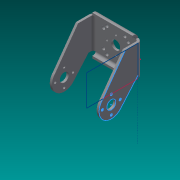
# Autodesk Inventor part: 45angle
Saved by Autodesk Inventor 2013 SP2 (Build 170200200, 200)
## iProperties
Created: 2014-11-26
Part Number: 45angle
Material: Generic
Document SubType Name: Sheet Metal
Designer: Master
Density: 1 g/cm^3
Sheet Metal Rule: Default_mm
Author: Master
Autodesk Inventor part; units mm, degrees
ref_plane "YZ Plane" through (0, 0, 0) normal (1, 0, 0) x (0, 1, 0)
ref_plane "XZ Plane" through (0, 0, 0) normal (0, 1, 0) x (-1, 0, 0)
ref_plane "XY Plane" through (0, 0, 0) normal (0, 0, 1) x (1, 0, 0)
sketch "Sketch1" plane through (0, 0, 0) normal (0, 1, 0) x (-1, 0, 0)
  circle A0 centre (0, 0) radius 4
  circle A1 centre (0, 8) radius 1
  circle A2 centre (8, 0) radius 1
  circle A3 centre (-8, 0) radius 1
  circle A4 centre (0, -8) radius 1
  circle A5 centre (-11, 8) radius 1.5
  circle A6 centre (11, -8) radius 1.5
  circle A7 centre (11, 8) radius 1.5
  circle A8 centre (-11, -8) radius 1.5
  line L0 (-18, 13.75) -> (18, 13.75)
  line L1 (18, 13.75) -> (18, -13.75)
  line L2 (18, -13.75) -> (-18, -13.75)
  line L3 (-18, -13.75) -> (-18, 13.75)
  line L4 (-17, 13.75) -> (19, -13.75) construction
  line L5 (19, 13.75) -> (-17, -13.75) construction
  point P0 (0, 0)
  dimension "d0" = 36
  dimension "d1" = 27.5
  measures "d0" distance of L1.end L2.end
  measures "d1" distance of L0.end L1.end
extrude "Plate1" add sketch "Sketch1" along normal blind 2
sketch "Sketch4" plane through (20, -2, 13.75) normal (1, 0, 0) x (0, 1, 0)
  line L0 (0, -27.5) -> (0, 0)
  line L1 (0, 0) -> (-46, 0)
  line L2 (-46, 0) -> (-46, -27.5)
  line L3 (-46, -27.5) -> (0, -27.5)
  constraints: 6 end point, 1 horizontal, 1 perpendicular, 1 vertical
edge flange "Flange3" height 50 angle 90 thickness 2 bend radius 2 thickness toward (1, 0, 0) relief straight relief width 2 relief depth 1 edges at (18, 0, 0) wall of the first edge with corners at (20, -2, -13.75) (20, -2, 13.75) (20, -48, 13.75) (20, -48, -13.75)
bend "Bend3"
corner "Corner3"
sketch "Sketch5" plane through (-20, -2, -13.75) normal (-1, 0, 0) x (0, -1, 0)
  line L0 (0, 27.5) -> (0, 0)
  line L1 (0, 0) -> (46, 0)
  line L2 (46, 0) -> (46, 27.5)
  line L3 (46, 27.5) -> (0, 27.5)
  constraints: 6 end point, 1 horizontal, 1 perpendicular, 1 vertical
edge flange "Flange4" height 50 angle 90 thickness 2 bend radius 2 thickness toward (-1, 0, 0) relief straight relief width 2 relief depth 1 edges at (-18, 0, 0) wall of the first edge with corners at (-20, -2, 13.75) (-20, -2, -13.75) (-20, -48, -13.75) (-20, -48, 13.75)
bend "Bend4"
corner "Corner4"
sketch "Sketch6" plane through (22, -48, 13.75) normal (1, 0, 0) x (0, 0, -1)
  line L0 (27.5, 46) -> (0, 46) projected
  line L1 (0, 0) -> (0, 46) projected
  line L2 (13.75, 46) -> (78.0909, 46) construction
  circle A0 centre (27.7916, 21.9584) radius 1
  circle A1 centre (35.7916, 29.9584) radius 1
  circle A2 centre (43.7916, 21.9584) radius 1
  circle A3 centre (35.7916, 13.9584) radius 1
  circle A4 centre (35.7916, 21.9584) radius 4
  arc A5 (28.0135, 14.1802) -> (42.3794, 30.7675) centre (35.7916, 21.9584) ccw
  line L3 (43.5698, 29.7365) -> (24.7916, 46)
  line L4 (28.0135, 14.1802) -> (0, 34.3911)
  line L5 (24.7916, 46) -> (27.5, 46)
  line L6 (24.7916, 46) -> (0, 46)
  line L7 (0, 46) -> (0, 34.3911)
  line L8 (27.5, 46) -> (27.5, 0) projected
  line L9 (0, 34.3911) -> (0, 0)
  line L10 (27.5, 0) -> (0, 0)
  line L11 (27.5, 0) -> (27.5, 14.5506)
  line L12 (27.5, 14.5506) -> (0, 34.3911)
  point P0 (13.75, 48)
  constraints: 20 end point, 6 centre point, 5 point on line, 4 collinear, 3 point on circle, 1 horizontal, 1 midpoint, 1 parallel, 1 perpendicular
sheet face with bend "Face2" sketch "Sketch6" thickness 2 toward (-1, 0, 0) bend radius 2 relief straight relief width 2 relief depth 1 contours L3 L8 A0 L4 L1 L0 | L3 A5 L4 L8 A0
bend "Bend5"
extrude "Cut1" cut sketch "Sketch6" against normal blind 2 contours L4 L8 L10 L1
sketch "Sketch7" plane through (0, 2, 0) normal (0, 1, 0) x (1, 0, 0)
  circle A0 centre (0, 0) radius 4 projected
  circle A1 centre (-11, -8) radius 1.5 projected
  circle A2 centre (11, -8) radius 1.5 projected
  circle A3 centre (-11, 8) radius 1.5 projected
  circle A4 centre (11, 8) radius 1.5 projected
  circle A5 centre (0, -8) radius 1 projected
  circle A6 centre (-8, 0) radius 1 projected
  circle A7 centre (8, 0) radius 1 projected
  circle A8 centre (0, 8) radius 1 projected
  line L0 (18, 11.75) -> (-18, 11.75) projected
  line L1 (-18, -13.75) -> (-18, 13.75) projected
  line L2 (-18, -11.75) -> (18, -11.75) projected
  line L3 (18, 13.75) -> (18, -13.75) projected
  line L4 (0, -11.75) -> (0, 11.75)
  constraints: 2 end point, 2 midpoint
ref_plane "Work Plane1" through (0, 2, 11.75) normal (1, 0, 0) x (0, 0, -1)
mirror "Mirror1" about plane through (0, 2, 11.75) normal (1, 0, 0) of "Flange3", "Face2"
sketch "Sketch8" plane through (-22, -48, -13.75) normal (-1, 0, 0) x (0, 0, 1)
  line L0 (0, 0) -> (0, 14.5506) projected
  line L1 (27.5, 0) -> (0, 0) projected
  line L2 (27.5, 46) -> (27.5, 0) projected
  line L3 (-0.5135, 14.1802) -> (27.5, 34.3911) projected
  line L4 (0, 14.5506) -> (27.5, 34.3911)
  line L5 (27.5, 34.3911) -> (27.5, 0)
  line L6 (0, 0) -> (0, 14.5506)
  line L7 (0, 0) -> (27.5, 0)
  point P0 (13.75, 48)
  constraints: 8 end point, 4 collinear
extrude "Cut2" cut sketch "Sketch8" against normal blind 2
sketch "Sketch9" plane through (0, 2, 0) normal (0, 1, 0) x (1, 0, 0)
  circle A0 centre (0, 0) radius 4 projected
  circle A1 centre (-11, -8) radius 1.5 projected
  circle A2 centre (11, -8) radius 1.5 projected
  circle A3 centre (-11, 8) radius 1.5 projected
  circle A4 centre (11, 8) radius 1.5 projected
  circle A5 centre (0, -8) radius 1 projected
  circle A6 centre (-8, 0) radius 1 projected
  circle A7 centre (8, 0) radius 1 projected
  circle A8 centre (0, 8) radius 1 projected
  line L0 (18, 11.75) -> (-18, 11.75) projected
  line L1 (-18, -13.75) -> (-18, 13.75) projected
  line L2 (-18, -11.75) -> (18, -11.75) projected
  line L3 (18, 13.75) -> (18, -13.75) projected
  line L4 (0, -4) -> (0, 4)
  constraints: 2 end point, 2 point on circle, 1 parallel
sketch "Sketch10" plane through (0, 2, 0) normal (0, 1, 0) x (1, 0, 0)
  circle A0 centre (0, 0) radius 4 projected
  circle A1 centre (-11, -8) radius 1.5 projected
  circle A2 centre (11, -8) radius 1.5 projected
  circle A3 centre (-11, 8) radius 1.5 projected
  circle A4 centre (11, 8) radius 1.5 projected
  circle A5 centre (0, -8) radius 1 projected
  circle A6 centre (-8, 0) radius 1 projected
  circle A7 centre (8, 0) radius 1 projected
  circle A8 centre (0, 8) radius 1 projected
  line L0 (18, 11.75) -> (-18, 11.75) projected
  line L1 (-18, -13.75) -> (-18, 13.75) projected
  line L2 (-18, -11.75) -> (18, -11.75) projected
  line L3 (18, 13.75) -> (18, -13.75) projected
sketch "Sketch11" plane through (0, 2, 0) normal (0, 1, 0) x (1, 0, 0)
  circle A0 centre (0, 0) radius 4 projected
  circle A1 centre (11, 8) radius 1.5 projected
  circle A2 centre (-11, 8) radius 1.5 projected
  circle A3 centre (11, -8) radius 1.5 projected
  circle A4 centre (-11, -8) radius 1.5 projected
  circle A5 centre (-11, 8) radius 1.5
  circle A6 centre (11, 8) radius 1.5
  circle A7 centre (11, -8) radius 1.5
  circle A8 centre (-11, -8) radius 1.5
  line L0 (8, -11) -> (-8, 11) construction
  line L1 (-8, -11) -> (8, 11) construction
  circle A9 centre (-8, 11) radius 1.5
  circle A10 centre (8, 11) radius 1.5
  circle A11 centre (8, -11) radius 1.5
  circle A12 centre (-8, -11) radius 1.5
  dimension "d62" = 16
  dimension "d63" = 22
  dimension "d64" = 3
  dimension "d65" = 3
  dimension "d66" = 3
  dimension "d67" = 3
  constraints: 8 centre point, 8 coincident, 4 end point, 2 midpoint, 1 concentric
  measures "d62" distance of L0.end L1.end
  measures "d63" distance of L1.start L0.end
  measures "d64" diameter of A9
  measures "d65" diameter of A10
  measures "d66" diameter of A11
  measures "d67" diameter of A12
extrude "Cut3" cut sketch "Sketch11" against normal blind 2 contours A9 | A10 | A11 | A12
sketch "Sketch12" plane through (-18, -2, 15.75) normal (0, 0, 1) x (1, 0, 0)
  line L0 (36, 0) -> (0, 0)
  line L1 (0, 0) -> (0, -1)
  line L2 (0, -1) -> (36, -1)
  line L3 (36, -1) -> (36, 0)
  constraints: 6 end point, 1 horizontal, 1 perpendicular, 1 vertical
edge flange "Flange5" height 5 angle 90 thickness 2 bend radius 2 thickness toward (0, 0, 1) relief straight relief width 2 relief depth 1 edges at (0, 0, 13.75) wall of the first edge with corners at (18, -2, 15.75) (-18, -2, 15.75) (-18, -3, 15.75) (18, -3, 15.75)
bend "Bend6"
corner "Corner5"
sketch "Sketch13" plane through (18, -2, -15.75) normal (0, 0, -1) x (-1, 0, 0)
  line L0 (36, 0) -> (0, 0)
  line L1 (0, 0) -> (0, -1)
  line L2 (0, -1) -> (36, -1)
  line L3 (36, -1) -> (36, 0)
  constraints: 6 end point, 1 horizontal, 1 perpendicular, 1 vertical
edge flange "Flange6" height 5 angle 90 thickness 2 bend radius 2 thickness toward (0, 0, -1) relief straight relief width 2 relief depth 1 edges at (0, 0, -13.75) wall of the first edge with corners at (-18, -2, -15.75) (18, -2, -15.75) (18, -3, -15.75) (-18, -3, -15.75)
bend "Bend7"
corner "Corner6"
equation "\"d51\" = Thickness"
equation "\"d54\" = Thickness"
equation "\"d68\" = Thickness"
equation "\"d23\" = BendReliefWidth"
equation "\"d24\" = BendReliefDepth"
equation "\"d25\" = MinimumRemnant"
equation "\"d26\" = BendRadius"
equation "\"d29\" = BendRadius"
equation "\"d30\" = CornerReliefSize"
equation "\"d31\" = GapSize"
equation "\"d32\" = JacobiRadiusSize"
equation "\"d33\" = BendReliefWidth"
equation "\"d34\" = BendReliefDepth"
equation "\"d35\" = MinimumRemnant"
equation "\"d36\" = BendRadius"
equation "\"d39\" = BendRadius"
equation "\"d40\" = CornerReliefSize"
equation "\"d41\" = GapSize"
equation "\"d42\" = JacobiRadiusSize"
equation "\"d46\" = BendRadius"
equation "\"d47\" = BendReliefWidth"
equation "\"d49\" = MinimumRemnant"
equation "\"d48\" = BendReliefDepth"
equation "\"d50\" = BendRadius"
equation "\"d70\" = BendReliefWidth"
equation "\"d71\" = BendReliefDepth"
equation "\"d72\" = MinimumRemnant"
equation "\"d73\" = BendRadius"
equation "\"d76\" = BendRadius"
equation "\"d77\" = CornerReliefSize"
equation "\"d78\" = GapSize"
equation "\"d79\" = JacobiRadiusSize"
equation "\"d80\" = BendReliefWidth"
equation "\"d81\" = BendReliefDepth"
equation "\"d82\" = MinimumRemnant"
equation "\"d83\" = BendRadius"
equation "\"d86\" = BendRadius"
equation "\"d87\" = CornerReliefSize"
equation "\"d88\" = GapSize"
equation "\"d89\" = JacobiRadiusSize"
equation "\"BendRadius\" = Thickness"
equation "\"BendReliefWidth\" = Thickness"
equation "\"BendReliefDepth\" = 0.5 * Thickness"
equation "\"CornerReliefSize\" = 4 * Thickness"
equation "\"MinimumRemnant\" = 2 * Thickness"
equation "\"TransitionRadius\" = BendRadius"
equation "\"JacobiRadiusSize\" = BendRadius"
equation "\"GapSize\" = Thickness"
equation "\"d2\" = BendRadius"
equation "\"Thickness\" = 2"
body "Solid1"
